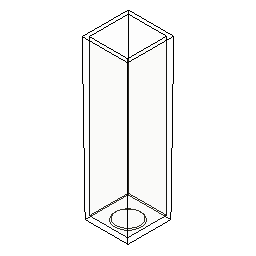
photometer_v0.1 (Autodesk Fusion 360 archive; units mm, degrees)
design "cuvette"
Autodesk Fusion 360 part; units mm, degrees
sketch "Sketch1" plane through (0, 0, 0) normal (0, 0, 1) x (1, 0, 0)
  line L0 (6, 6) -> (-6, 6)
  line L1 (-6, 6) -> (-6, -6)
  line L2 (-6, -6) -> (6, -6)
  line L3 (6, -6) -> (6, 6)
  line L4 (6, 6) -> (-6, -6) construction
  line L5 (-6, 6) -> (6, -6) construction
  circle A0 centre (0, 0) radius 3.65
  dimension "d1" = 12
  dimension "d2" = 12
  dimension "d9" = 7.3
  constraint horizontal L0
  constraint perpendicular L0 L1
  constraint parallel L0 L2
  constraint parallel L1 L3
  constraint coincident L4 A0.centre
  constraint coincident L5 A0.centre
  constraint coincident A0.centre origin
  measures "d1" distance of L1.end L2.end
  measures "d2" distance of L0.end L1.end
  measures "d9" diameter of A0
ref_plane "WorkPlane1" through (0, 0, 44.4) normal (0, 0, 1) x (1, 0, 0)
sketch "Sketch2" plane through (0, 0, 44.4) normal (0, 0, 1) x (1, 0, 0)
  line L0 (6.35, 6.45) -> (-6.35, 6.45)
  line L1 (-6.35, 6.45) -> (-6.35, -6.45)
  line L2 (-6.35, -6.45) -> (6.35, -6.45)
  line L3 (6.35, -6.45) -> (6.35, 6.45)
  line L4 (6.35, 6.45) -> (-6.35, -6.45) construction
  line L5 (-6.35, 6.45) -> (6.35, -6.45) construction
  line L6 (-5.35, -5.45) -> (5.35, -5.45)
  line L7 (5.35, -5.45) -> (5.35, 5.45)
  line L8 (5.35, 5.45) -> (-5.35, 5.45)
  line L9 (-5.35, 5.45) -> (-5.35, -5.45)
  dimension "d4" = 12.7
  dimension "d5" = 12.9
  dimension "d6" = -1
  constraint horizontal L0
  constraint perpendicular L0 L1
  constraint parallel L0 L2
  constraint parallel L1 L3
  constraint coincident L4 origin
  constraint coincident L5 origin
  measures "d4" distance of L1.end L2.end
  measures "d5" distance of L0.end L1.end
loft "Loft1" add profiles "Sketch1", "Sketch2" section 1 contours L0 L1 L2 L3 | A0 section 2 contours L0 L1 L2 L3 | L6 L7 L8 L9
extrude "Extrude1" cut sketch "Sketch2" against normal blind 43.4 contours L6 L7 L8 L9
extrude "Extrude2" cut sketch "Sketch1" along normal blind 0.25 contours A0
fillet "Fillet1" radius 0.3 1 edges at (-3.403, -1.3199, 0.25)

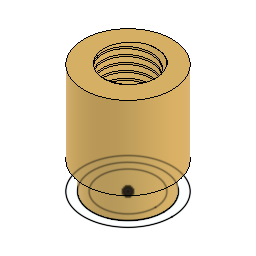
design "threaded_m2_brass_insert"
Autodesk Fusion 360 part; units mm, degrees
sketch "Sketch1" plane through (0, 0, 0) normal (0, 0, 1) x (1, 0, 0)
  circle A0 centre (0, 0) radius 1.3
  circle A1 centre (0, 0) radius 1.6
  circle A2 centre (0, 0) radius 1
  dimension "d1" = 2.6
  dimension "d2" = 3.2
  dimension "d3" = 2
  constraint coincident A0.centre A1.centre
  constraint concentric A0 A2
  measures "d1" diameter of A0
  measures "d2" diameter of A1
  measures "d3" diameter of A2
extrude "Extrude1" add sketch "Sketch1" along normal blind 4 contours A0
extrude "Extrude2" add sketch "Sketch1" along normal blind 3 from surface at 1 contours A1
thread "Thread1" "ISO Metric profile 2.0 M2x0.25 M2x0.25 6H" major diameter 2.0555 minor diameter 1.7694 pitch 0.25 angle 60 modelled right hand crest width 0.064 on face at (0.9988, -0.0498, 2.6667) crest through (0.8847, 0, 0.0625)

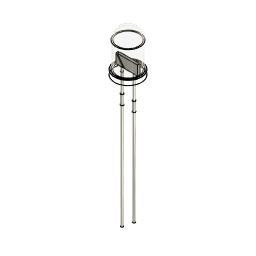
design "F3D_LED_DIODE_5mm"
Autodesk Fusion 360 part; units mm, degrees
sketch "Sketch1" plane through (0, 0, 0) normal (0, 1, 0) x (1, 0, 0)
  line L0 (0, 0) -> (2.5, 0)
  line L1 (2.5, 0) -> (2.5, -8.8)
  line L2 (2.5, -8.8) -> (0, -8.8)
  line L3 (0, -8.8) -> (0, 0)
  line L4 (2.5, 0) -> (2.8, 0)
  line L5 (2.8, 0) -> (2.8, -1)
  line L6 (2.8, -1) -> (2.5, -1)
  line L7 (2.5, -1) -> (2.5, 0)
  circle A0 centre (0, -6.3) radius 2.5
  circle A1 centre (0, -6.3) radius 2.25
  line L8 (2.25, -6.3) -> (2.25, 0)
  line L9 (2.25, -1) -> (0, -1)
  line L10 (0, -1) -> (0, 0)
  line L11 (0, 0) -> (2.25, 0)
  line L12 (2.25, 0) -> (2.25, -1)
  dimension "d1" = 8.8
  dimension "d2" = 2.5
  dimension "d3" = 2.8
  dimension "d4" = 1
  dimension "d5" = 5
  dimension "d6" = 4.5
  constraint horizontal L0
  constraint vertical L1
  constraint horizontal L2
  constraint vertical L3
  constraint coincident L0.start L3.end
  constraint horizontal L4
  constraint vertical L5
  constraint horizontal L6
  constraint vertical L7
  constraint coincident L3 A0.centre
  constraint coincident L2.end A0
  constraint tangent L1 A0
  constraint concentric A0 A1
  constraint coincident A1 L8.start
  constraint coincident L0 L8.end
  constraint tangent A1 L8
  constraint perpendicular L0 L8
  constraint horizontal L9
  constraint vertical L10
  constraint horizontal L11
  constraint vertical L12
  constraint coincident L8 L9.start
  measures "d1" distance of L0.end L1.end
  measures "d2" distance of L1.end L2.end
  measures "d3" distance of L3 L5
  measures "d4" distance of L4.end L5.end
  measures "d5" diameter of A0
  measures "d6" diameter of A1
revolve "Revolve1" add sketch "Sketch1" angle 360 about axis through (0, 0, 8.8) along (0, 0, -1) contours L0 L3 L8 L9 L10 L11 L12 | L0 L1 L7 A0 L8 L12 | L1 L4 L5 L6 L7 | L3 A0 A1 L8 picked at (0.5647, -8.644) makes body 1
sketch "Sketch2" plane through (0, 0, 0) normal (0, 1, 0) x (1, 0, 0)
  line L0 (-2.25, -6.3) -> (2.25, -6.3)
  line L1 (-2.25, -1) -> (2.25, -1)
  line L2 (-2.25, -1) -> (-2.25, -3)
  line L3 (-2.25, -3) -> (-0.75, -1)
  line L4 (-1.9375, -3) -> (2.25, -3)
  line L5 (2.25, -3) -> (2.25, -1)
  line L6 (-0.4375, -1) -> (-1.9375, -3)
  dimension "d8" = 2
  dimension "d9" = 1.5
  dimension "d10" = 0.25
  constraint coincident L1.start L2.start
  constraint perpendicular L1 L2
  constraint coincident L1 L3.end
  constraint perpendicular L2 L4
  constraint coincident L1.end L5.end
  constraint perpendicular L1 L5
  constraint coincident L1 L6.start
  constraint parallel L3 L6
  constraint horizontal L2.end L4.start
  measures "d8" distance of L1.start L2.end
  measures "d9" distance of L2 L3.end
  measures "d10" distance of L3 L6
extrude "Extrude1" add sketch "Sketch2" along normal mid plane 0.5 separate body makes body 2 at (-1.75, 0.25, 1.6667) makes body 3 at (-0.0417, 0.25, 2.3333)
sketch "Sketch3" plane through (0, 0, 1) normal (0, 0, -1) x (1, 0, 0)
  line L0 (-2.25, 0.25) -> (-2.25, -0.25)
  line L1 (-2.25, -0.25) -> (-0.75, -0.25)
  line L2 (-0.75, -0.25) -> (-0.75, 0.25)
  line L3 (-0.75, 0.25) -> (-2.25, 0.25)
  circle A0 centre (-1.25, 0) radius 0.25
  circle A1 centre (1.25, 0) radius 0.25
  line L4 (-0.4375, 0.25) -> (2.25, 0.25)
  dimension "d13" = 1.25
  dimension "d14" = 1.25
  dimension "d15" = 0.5
  constraint tangent L1 A0
  constraint tangent L3 A0
  constraint horizontal origin A1.centre
  constraint tangent A1 L4
  measures "d13" distance of origin A0.centre
  measures "d14" distance of origin A1.centre
  measures "d15" diameter of A0
extrude "Extrude2" cut sketch "Sketch3" along normal blind 1.6 contours A0 | A1 bodies 1
extrude "Extrude3" add sketch "Sketch3" along normal blind 29 contours A0 bodies 2
extrude "Extrude4" add sketch "Sketch3" along normal blind 27 contours A1 bodies 3
fillet "Fillet1" radius 0.03 1 edges at (-2.3308, -0.904, 1) 1 faces at (2.7965, 0.1396, 0.3333) on bodies 1
fillet "Fillet2" radius 0.04 2 faces at (-1.3097, -0.1688, -28) (1.1749, -0.1495, -26) on bodies 2 3
sketch "Sketch4" plane through (0, 0, 0) normal (0, 1, 0) x (1, 0, 0)
  line L0 (-1, -1) -> (-1, 27.96)
  line L1 (-1.5, 27.96) -> (-1.5, -1)
  line L2 (1.5, -1) -> (1.5, 25.96)
  line L3 (1, 25.96) -> (1, -1)
  line L4 (-1, 4) -> (-0.95, 4)
  line L5 (-0.95, 4) -> (-0.95, 6)
  line L6 (-0.95, 6) -> (-1, 6)
  line L7 (-1, 6) -> (-1, 4)
  line L8 (1.5, 4) -> (1.55, 4)
  line L9 (1.55, 4) -> (1.55, 6)
  line L10 (1.55, 6) -> (1.5, 6)
  line L11 (1.5, 6) -> (1.5, 4)
  line L12 (-2.77, 0) -> (2.77, 0)
  dimension "d26" = 4
  dimension "d27" = 2
  dimension "d28" = 0.05
  dimension "d29" = 0.05
  constraint horizontal L4
  constraint vertical L5
  constraint horizontal L6
  constraint vertical L7
  constraint coincident L0 L4.start
  constraint horizontal L8
  constraint vertical L9
  constraint horizontal L10
  constraint vertical L11
  constraint coincident L2 L8.start
  constraint horizontal L5.end L9.end
  constraint horizontal L4.end L8.end
  measures "d26" distance of L4 L12
  measures "d27" distance of L8.end L9.end
  measures "d28" distance of L8.start L8.end
  measures "d29" distance of L4.start L4.end
revolve "Revolve2" add sketch "Sketch4" angle 360 about axis through (-1.25, 0, 1) along (0, 0, 1) contours L0 L4 L5 L6 L7 bodies 2
revolve "Revolve3" add sketch "Sketch4" angle 360 about axis through (1.25, 0, 1) along (0, 0, 1) contours L2 L8 L9 L10 L11 bodies 3
fillet "Fillet3" radius 0.01 4 faces at (-0.9678, -0.0149, -4) (-0.9687, -0.0273, -6) (1.5322, -0.0149, -4) (1.5313, -0.0273, -6) on bodies 2 3
sketch "Sketch5" plane through (0, 0, 0) normal (1, 0, 0) x (0, 1, 0)
  circle A0 centre (0.6836, 1.8962) radius 0.3321
  line L0 (0.6836, 2.2284) -> (0.6836, 1.5641)
  constraint coincident A0 L0.start
  constraint coincident A0 L0.end
  constraint vertical L0
revolve "Revolve4" add sketch "Sketch5" angle 360 about axis through (0, 0.6836, 2.2284) along (0, 0, -1) separate body contours A0 L0 picked at (0.7673, 1.9687) makes body 4
hidden bodies 4
equation "d2 = ( 5 / 2 ) * 1 mm"
equation "d3 = ( 5.6 / 2 ) * 1 mm"
equation "d6 = d5 - 0.5 mm"
equation "d11 = ( 0.5 / 2 ) * 1 mm"
equation "d13 = 1 mm + d15 / 2"
equation "d14 = d13"
equation "d29 = d28"
named bodies: "LED DIODE CAP", "LED FILAMENT", "LED LEGS"
